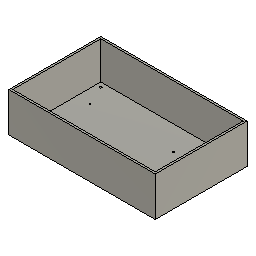
Ensamble Caja con Fuente (Autodesk Fusion 360 archive; units mm, degrees)
design "Caja_Base"
Autodesk Fusion 360 part; units mm, degrees
note: some values were not read from the file. Set by a fixed rule: which face or edge a step refers to.
sketch "Sketch1" plane through (0, 0, 0) normal (0, 0, 1) x (1, 0, 0)
  line L0 (0, 0) -> (223, 0)
  line L1 (223, 0) -> (223, 140)
  line L2 (223, 140) -> (0, 140)
  line L3 (0, 140) -> (0, 0)
  dimension "d1" = 223
  dimension "d2" = 140
  constraint horizontal L0
  constraint vertical L1
  constraint horizontal L2
  constraint vertical L3
  constraint coincident L0.start L3.end
  measures "d1" distance of L0.start L0.end
  measures "d2" distance of L0.end L1.end
extrude "Extrude1" add sketch "Sketch1" along normal blind 20
shell "Shell1" thickness 3 removed faces 1 at (74.3333, 93.3333, 20)
sketch "Sketch2" plane through (0, 0, 0) normal (0, 0, -1) x (1, 0, 0)
  line L0 (0, 0) -> (0, -140)
  line L1 (0, -140) -> (223, -140)
  line L2 (223, -140) -> (223, 0)
  line L3 (223, 0) -> (0, 0)
  circle A0 centre (151.0199, -99.7985) radius 1.25
  line L4 (211.0199, -114.4985) -> (211.0199, -5.5017) construction
  line L5 (12.0134, -5.5017) -> (12.0134, -114.4985) construction
  line L6 (211.0199, -60) -> (157.0519, -60) construction
  circle A1 centre (24.0134, -99.7985) radius 1.25
  circle A2 centre (24.0134, -20.2015) radius 1.25
  circle A3 centre (151.0199, -20.2015) radius 1.25
  line L7 (12.0134, -114.4985) -> (211.0199, -114.4985) construction
  line L8 (211.0199, -114.4985) -> (15.7448, -114.4985) construction
  line L9 (211.0199, -5.5017) -> (12.0134, -5.5017) construction
  circle A4 centre (10, -130) radius 1.5
  circle A5 centre (213, -130) radius 1.5
  line L10 (210, -70) -> (223, -70) construction
  circle A6 centre (10, -10) radius 1.5
  circle A7 centre (213, -10) radius 1.5
  point P0 (190.3238, -109.2905)
  dimension "d7" = 14.7
  dimension "d8" = 2.5
  dimension "d9" = 108.9968
  dimension "d10" = 54.4985
  dimension "d11" = 2.5
  dimension "d12" = 60
  dimension "d13" = 14.7
  dimension "d15" = 3
  dimension "d16" = 10
  dimension "d17" = 10
  dimension "d18" = 10
  dimension "d19" = 10
  dimension "d20" = 3
  dimension "d21" = 70
  dimension "d24" = 80
  dimension "d27" = 199.0065
  constraint coincident L4.start L7.end
  constraint coincident L6.start L4
  constraint perpendicular L4 L6
  constraint symmetric L6 A1 A2
  constraint symmetric A0 L6 A3
  constraint coincident L2 L10.end
  constraint perpendicular L2 L10
  constraint symmetric A4 L10 A6
  constraint symmetric A5 L10 A7
  measures "d7" distance of A1.centre L8
  measures "d8" diameter of A1
  measures "d9" distance of L7 L9
  measures "d10" distance of L6 L7
  measures "d11" diameter of A0
  measures "d12" distance of A0.centre L4
  measures "d13" distance of A0.centre L7
  measures "d15" diameter of A4
  measures "d16" distance of L0 A4.centre
  measures "d17" distance of L1 A4.centre
  measures "d18" distance of L2 A5.centre
  measures "d19" distance of L1 A5.centre
  measures "d20" diameter of A5
  measures "d21" distance of L1 L10
  measures "d24" distance of L1 L6
  measures "d27" distance of L4 L5
extrude "Extrude2" cut sketch "Sketch2" against normal up to surface (3 mm away) contours A0 | A1 | A2 | A3 | A4 | A5 | A6 | A7
extrude "Extrude3" add 1 faces at (75.3333, 1, 20) along direction (0, 0, 1) blind 40
equation "d21 = ( 140 / 2 ) * 1 mm"
